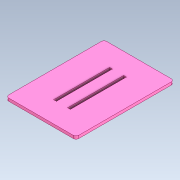
# Autodesk Inventor part: Base
Saved by Autodesk Inventor 2021 (Build 250183000, 183)
## iProperties
Created: 2021-08-28
Part Number: Base
Material: ABS Plastic
Document SubType Name: Modeling
Designer: digge
Density: 1.06 g/cm^3
Appearance: Pink
Author: digge
Autodesk Inventor part; units mm, degrees
ref_plane "YZ Plane" through (0, 0, 0) normal (1, 0, 0) x (0, 1, 0)
ref_plane "XZ Plane" through (0, 0, 0) normal (0, 1, 0) x (-1, 0, 0)
ref_plane "XY Plane" through (0, 0, 0) normal (0, 0, 1) x (1, 0, 0)
sketch "Sketch1" plane through (0, 0, 0) normal (0, 1, 0) x (-1, 0, 0)
  line L0 (104.6154, 153.8462) -> (-145.3846, 153.8462)
  line L1 (-145.3846, 153.8462) -> (-145.3846, -196.1538)
  line L2 (-145.3846, -196.1538) -> (104.6154, -196.1538)
  line L3 (104.6154, -196.1538) -> (104.6154, 153.8462)
  line L4 (-20.3846, 153.8462) -> (-20.3846, -196.1538) construction
  line L5 (104.6154, -21.1538) -> (-145.3846, -21.1538) construction
  line L6 (9.6154, 78.8462) -> (-0.3846, 78.8462)
  line L7 (-0.3846, 78.8462) -> (-0.3846, -121.1538)
  line L8 (-0.3846, -121.1538) -> (9.6154, -121.1538)
  line L9 (9.6154, -121.1538) -> (9.6154, 78.8462)
  line L10 (-40.3846, 78.8462) -> (-50.3846, 78.8462)
  line L11 (-50.3846, 78.8462) -> (-50.3846, -121.1538)
  line L12 (-50.3846, -121.1538) -> (-40.3846, -121.1538)
  line L13 (-40.3846, -121.1538) -> (-40.3846, 78.8462)
  point P0 (0, 0)
  dimension "d0" = 250
  dimension "d1" = 350
  dimension "d2" = 10
  dimension "d3" = 10
  dimension "d4" = 200
  dimension "d7" = 40
  constraints: 28 end point, 6 parallel, 4 midpoint, 3 horizontal, 3 perpendicular, 2 collinear, 2 other
  measures "d0" distance of L0.start L0.end
  measures "d1" distance of L2.end L0.start
  measures "d2" distance of L10.start L10.end
  measures "d3" distance of L6.start L6.end
  measures "d4" distance of L8.end L6.start
  measures "d7" distance between parallel lines of L13 L7
extrude "Extrusion1" add sketch "Sketch1" along normal blind 10
fillet "Fillet1" radius 10 4 edges at (145.3846, 5, -196.1538) (-104.6154, 5, -196.1538) (-104.6154, 5, 153.8462) (145.3846, 5, 153.8462)
equation "\"d0\" = BaseDepth"
equation "\"d1\" = BaseLength"
equation "\"d2\" = Width"
equation "\"d3\" = Width"
equation "\"d4\" = SlotLength"
equation "\"d7\" = 4 * Width"
equation "\"d5\" = Width"
equation "\"BaseDepth\" = 250"
equation "\"BaseLength\" = 350"
equation "\"Width\" = 10"
equation "\"SlotLength\" = 200"
body "Solid1"
